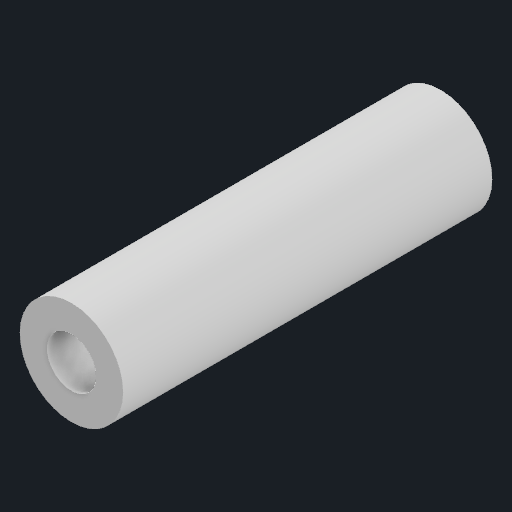
# Autodesk Inventor part: ptfe filament guide
Saved by Autodesk Inventor 2024.3 (Build 283343000, 343)
## iProperties
Created: 2024-09-28
Part Number: ptfe filament guide
Material: Generic
Document SubType Name: Modeling
Designer: MFil
Density: 1 g/cm^3
Appearance: Default
Author: MFil
Autodesk Inventor part; units mm, degrees
ref_plane "YZ Plane" through (0, 0, 0) normal (1, 0, 0) x (0, 1, 0)
ref_plane "XZ Plane" through (0, 0, 0) normal (0, 1, 0) x (-1, 0, 0)
ref_plane "XY Plane" through (0, 0, 0) normal (0, 0, 1) x (1, 0, 0)
sketch "Sketch1" plane through (0, 0, 0) normal (0, 0, 1) x (1, 0, 0)
  circle A0 centre (2.042, 0) radius 0.875 projected
  circle A1 centre (2.042, 0) radius 2.1
  circle A2 centre (2.042, 0) radius 1
  point P0 (0, 0)
  dimension "d0" = 4.2
  dimension "d1" = 2
  constraints: 2 centre point, 2 coincident
  measures "d0" diameter of A1
  measures "d1" diameter of A2
extrude "Extrusion1" add sketch "Sketch1" along normal blind 12.5 and the other way blind 2.5 contours A1
body "Solid1"
